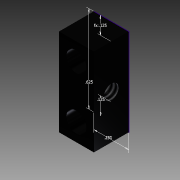
# Autodesk Inventor part: Cim Adjustment Block
Saved by Autodesk Inventor 2013 (Build 170138000, 138)
## iProperties
Created: 2013-06-28
Part Number: Cim Adjustment Block
Material: Generic
Document SubType Name: Modeling
Designer: mvarma
Density: 1 g/cm^3
Author: mvarma
Autodesk Inventor part; units mm, degrees
ref_plane "YZ Plane" through (0, 0, 0) normal (1, 0, 0) x (0, 1, 0)
ref_plane "XZ Plane" through (0, 0, 0) normal (0, 1, 0) x (-1, 0, 0)
ref_plane "XY Plane" through (0, 0, 0) normal (0, 0, 1) x (1, 0, 0)
sketch "Sketch1" plane through (0, 0, 0) normal (0, 0, 1) x (1, 0, 0)
  line L0 (0, 0) -> (6.35, 0)
  line L1 (6.35, 0) -> (6.35, 15.875)
  line L2 (6.35, 15.875) -> (0, 15.875)
  line L3 (0, 15.875) -> (0, 0)
  line L4 (3.175, 15.875) -> (3.175, 0) construction
  point P0 (3.175, 12.7)
  point P1 (3.175, 3.175)
  dimension "d0" = 6.35
  dimension "d1" = 15.875
  dimension "d2" = 3.175
  dimension "d3" = 3.175
  constraints: 10 end point, 2 midpoint, 2 parallel, 2 point on line, 1 horizontal, 1 perpendicular, 1 vertical
  measures "d0" distance of L0.start L0.end
  measures "d1" distance of L2.end L0.start
  measures "d2" distance from line of L0 point (3.175, 3.175)
  measures "d3" distance from line of L2 point (3.175, 12.7)
extrude "Extrusion1" add sketch "Sketch1" along normal blind 6.35
hole "Hole1" at (3.175, 12.7, 0) at (3.175, 3.175, 0) direction (0, 0, 1) diameter 3.6576 end through all clearance for "Flat Head Machine Screw (82)" size "#6" standard "Ansi Unified Screw Threads"
sketch "Sketch2" plane through (0, 0, 0) normal (-1, 0, 0) x (0, 0, 1)
  line L0 (6.35, 15.875) -> (6.35, 0) projected
  line L1 (0, 15.875) -> (6.35, 15.875) projected
  point P0 (3.175, 7.9375)
  dimension "d13" = 3.175
  dimension "d14" = 7.9375
  measures "d13" distance from line of point (3.175, 7.938) L0
  measures "d14" distance from line of point (3.175, 7.938) L1
hole "Hole2" at (0, 7.9375, 3.175) direction (1, 0, 0) diameter 2.6416 end through all thread size "6-32 UNC" class "2B" standard "ANSI Unified Screw Threads"
equation "\"d3\" = d2"
body "Solid1"
